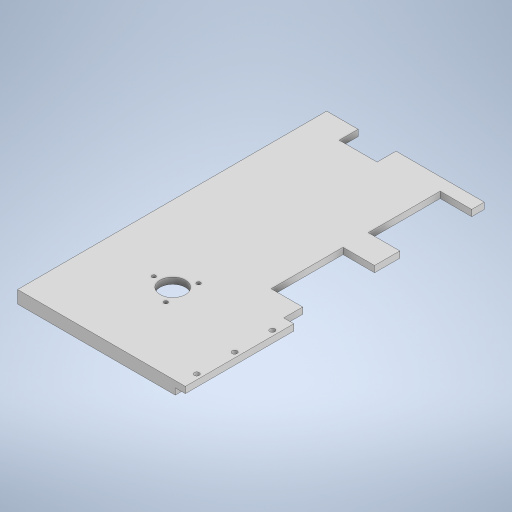
# Autodesk Inventor part: top_1
Saved by Autodesk Inventor 2023 (Build 270158000, 158)
## iProperties
Created: 2024-04-26
Part Number: top_1
Material: 常规
Document SubType Name: Modeling
Designer: Nitrene.P.L
Density: 1 g/cm^3
Appearance: 默认
Author: Nitrene.P.L
Autodesk Inventor part; units mm, degrees
ref_plane "YZ Plane" through (0, 0, 0) normal (1, 0, 0) x (0, 1, 0)
ref_plane "XZ Plane" through (0, 0, 0) normal (0, 1, 0) x (-1, 0, 0)
ref_plane "XY Plane" through (0, 0, 0) normal (0, 0, 1) x (1, 0, 0)
sketch "草图1" plane through (0, 0, 0) normal (0, 1, 0) x (-1, 0, 0)
  line L0 (125, 245) -> (-125, 245)
  line L1 (-125, 245) -> (-125, -245)
  line L2 (-125, -245) -> (125, -245)
  line L3 (125, -245) -> (125, 245)
  line L4 (0, 3) -> (0, -5)
  line L5 (3.5058, 0) -> (-3.4421, 0)
  circle A0 centre (621.9162, 528.0902) radius 10
  circle A1 centre (621.9162, 543.0902) radius 1.5
  circle A2 centre (634.9065, 520.5902) radius 1.5
  circle A3 centre (608.9258, 520.5902) radius 1.5
  line L6 (25, 144) -> (-32, 144)
  line L7 (-32, 144) -> (-32, 87)
  line L8 (-32, 87) -> (25, 87)
  line L9 (25, 87) -> (25, 144)
  line L10 (25, 67) -> (-32, 67)
  line L11 (-32, 67) -> (-32, 10)
  line L12 (-32, 10) -> (25, 10)
  line L13 (25, 10) -> (25, 67)
  line L14 (25, -10) -> (-32, -10)
  line L15 (-32, -10) -> (-32, -67)
  line L16 (-32, -67) -> (25, -67)
  line L17 (25, -67) -> (25, -10)
  line L18 (25, -87) -> (-32, -87)
  line L19 (-32, -87) -> (-32, -144)
  line L20 (-32, -144) -> (25, -144)
  line L21 (25, -144) -> (25, -87)
  line L22 (-66, 100) -> (-95, 100)
  line L23 (-95, 100) -> (-95, 54)
  line L24 (-95, 54) -> (-66, 54)
  line L25 (-66, 54) -> (-66, 100)
  line L26 (-66, -54) -> (-95, -54)
  line L27 (-95, -54) -> (-95, -100)
  line L28 (-95, -100) -> (-66, -100)
  line L29 (-66, -100) -> (-66, -54)
  line L30 (100, 15) -> (70, 15)
  line L31 (70, 15) -> (70, -15)
  line L32 (70, -15) -> (100, -15)
  line L33 (100, -15) -> (100, 15)
  circle A4 centre (65, 182) radius 10
  circle A5 centre (65, -182) radius 10
  circle A6 centre (65, 182) radius 15
  circle A7 centre (80, 182) radius 1.5
  circle A8 centre (57.5, 194.9904) radius 1.5
  circle A9 centre (57.5, 169.0096) radius 1.5
  line L34 (125, 245) -> (0, 245)
  line L35 (0, 245) -> (0, 0)
  line L36 (0, 0) -> (125, 0)
  line L37 (125, 0) -> (125, 245)
  line L38 (-125, 245) -> (0, 245)
  line L39 (0, 245) -> (0, 0)
  line L40 (0, 0) -> (-125, 0)
  line L41 (-125, 0) -> (-125, 245)
  line L42 (-125, -245) -> (0, -245)
  line L43 (0, -245) -> (0, 0)
  line L44 (0, 0) -> (-125, 0)
  line L45 (-125, 0) -> (-125, -245)
  line L46 (125, -245) -> (0, -245)
  line L47 (0, -245) -> (0, 0)
  line L48 (0, 0) -> (125, 0)
  line L49 (125, 0) -> (125, -245)
  point P0 (0, 87)
  point P1 (0, 67)
  point P2 (0, 10)
  point P3 (70, 0)
  point P4 (100, 0)
  point P5 (0, 144)
  dimension "d31" = 30
  dimension "d0" = 490
  dimension "d1" = 250
  dimension "d2" = 57
  dimension "d3" = 57
  dimension "d4" = 57
  dimension "d5" = 57
  dimension "d6" = 57
  dimension "d7" = 57
  dimension "d8" = 57
  dimension "d9" = 57
  dimension "d10" = 101
  dimension "d11" = 20
  dimension "d12" = 20
  dimension "d13" = 20
  dimension "d14" = 93
  dimension "d15" = 29
  dimension "d16" = 46
  dimension "d17" = 46
  dimension "d18" = 145
  dimension "d19" = 108
  dimension "d20" = 30
  dimension "d21" = 30
  dimension "d22" = 30
  dimension "d23" = 25
  dimension "d24" = 230
  dimension "d25" = 20
  dimension "d26" = 63
  dimension "d27" = 60
  dimension "d28" = 20
  dimension "d29" = 63
  dimension "d30" = 60
  dimension "d33" = 3
  dimension "d36" = 360
  constraints: 100 end point, 24 parallel, 14 horizontal, 12 perpendicular, 9 centre point, 3 collinear, 2 point on line, 2 vertical, 1 coincident, 1 horizontal alignment, 11 other
  measures "d0" distance of L2.end L0.start
  measures "d1" distance of L0.start L0.end
  measures "d2" distance of L8.end L7.end
  measures "d3" distance of L7.end L6.end
  measures "d4" distance of L12.end L11.end
  measures "d5" distance of L11.end L10.end
  measures "d6" distance of L16.end L15.end
  measures "d7" distance of L15.end L14.end
  measures "d8" distance of L20.end L19.end
  measures "d9" distance of L19.end L18.end
  measures "d10" distance between parallel lines of L0 L6
  measures "d11" distance between parallel lines of L10 L8
  measures "d12" distance between parallel lines of L12 L14
  measures "d13" distance between parallel lines of L18 L16
  measures "d14" distance between parallel lines of L1 L7
  measures "d15" distance of L24.end L23.end
  measures "d16" distance of L23.end L22.end
  measures "d17" distance of L27.end L26.end
  measures "d18" distance between parallel lines of L0 L22
  measures "d19" distance between parallel lines of L26 L24
  measures "d20" distance between parallel lines of L1 L23
  measures "d21" distance of L32.end L31.end
  measures "d22" distance of L31.end L30.end
  measures "d23" distance between parallel lines of L3 L33
  measures "d24" distance between parallel lines of L0 L30
  measures "d25" diameter of A4
  measures "d26" distance from line of L0 A4.centre
  measures "d27" distance from line of L3 A4.centre
  measures "d28" diameter of A5
  measures "d29" distance from line of L2 A5.centre
  measures "d30" distance from line of L3 A5.centre
  measures "d33" diameter of A7
extrude "拉伸1" add sketch "草图1" along normal blind 10 contours L3 L36 L33 L30 L31 L5 L4 L35 L12 L13 L10 L8 L9 L6 L0 | A7 A6 A9 A8
sketch "草图2" plane through (0, 0, 0) normal (0, -1, 0) x (1, 0, 0)
  line L0 (-100, 0) -> (-125, 0) projected
  line L1 (-115, 0) -> (-55, 0)
  line L2 (-55, 0) -> (-55, 30)
  line L3 (-55, 30) -> (-115, 30)
  line L4 (-115, 30) -> (-115, 0)
  line L5 (-100, 15) -> (-100, 0) projected
  line L6 (0, 0) -> (-70, 0) projected
  line L7 (0, 245) -> (0, 144) projected
  line L8 (-40, 0) -> (0, 0)
  line L9 (0, 0) -> (0, 159)
  line L10 (0, 159) -> (-40, 159)
  line L11 (-40, 159) -> (-40, 0)
  line L12 (-25, 67) -> (-25, 10) projected
  line L13 (0, 144) -> (-25, 144) projected
  circle A0 centre (-65, 182) radius 10 projected
  circle A1 centre (-65, 182) radius 20
  dimension "d40" = 60
  dimension "d41" = 30
  dimension "d42" = 15
  dimension "d43" = 15
  dimension "d44" = 15
  dimension "d45" = 40
  constraints: 16 end point, 4 parallel, 3 point on line, 2 horizontal, 2 perpendicular, 1 centre point, 1 coincident
  measures "d40" distance of L3.end L2.end
  measures "d41" distance of L2.end L1.end
  measures "d42" distance between parallel lines of L5 L4
  measures "d43" distance between parallel lines of L11 L12
  measures "d44" distance between parallel lines of L13 L10
  measures "d45" diameter of A1
extrude "拉伸2" cut sketch "草图2" against normal blind 5
sketch "草图3" plane through (0, 10, 0) normal (0, 1, 0) x (1, 0, 0)
  line L0 (-40, -159) -> (0, -159) projected
  line L1 (0, -159) -> (8, -159)
  line L2 (8, -159) -> (8, -245)
  line L3 (8, -245) -> (0, -245)
  line L4 (0, -245) -> (0, -159)
  circle A0 centre (4, -232) radius 2
  circle A1 centre (4, -202) radius 2
  circle A2 centre (4, -172) radius 2
  point P0 (0, 0)
  dimension "d48" = 4
  dimension "d49" = 4
  dimension "d50" = 4
  dimension "d51" = 30
  dimension "d52" = 30
  dimension "d53" = 13
  dimension "d54" = 4
  dimension "d55" = 4
  dimension "d56" = 4
  dimension "d57" = 8
  constraints: 8 end point, 3 centre point, 2 parallel, 1 horizontal, 1 perpendicular
  measures "d48" diameter of A0
  measures "d49" diameter of A1
  measures "d50" diameter of A2
  measures "d51" distance of A1.centre A0.centre
  measures "d52" distance of A1.centre A2.centre
  measures "d53" distance from line of L1 A2.centre
  measures "d54" distance from line of L4 A0.centre
  measures "d55" distance from line of L4 A1.centre
  measures "d56" distance from line of L4 A2.centre
  measures "d57" distance of L2.end L3.end
extrude "拉伸3" add sketch "草图3" against normal blind 5
